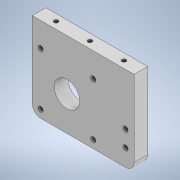
# Autodesk Inventor part: X-Axis_motor_plate
Saved by Autodesk Inventor 2021.3 (Build 253353000, 353)
## iProperties
Created: 2021-04-15
Part Number: X-Axis_motor_plate
Material: Generic
Document SubType Name: Modeling
Designer: Fabijan_Sven
Density: 1 g/cm^3
Appearance: Default
Author: Fabijan_Sven
Autodesk Inventor part; units mm, degrees
ref_plane "YZ Plane" through (0, 0, 0) normal (1, 0, 0) x (0, 1, 0)
ref_plane "XZ Plane" through (0, 0, 0) normal (0, 1, 0) x (-1, 0, 0)
ref_plane "XY Plane" through (0, 0, 0) normal (0, 0, 1) x (1, 0, 0)
sketch "Sketch1" plane through (0, 0, 0) normal (0, 1, 0) x (-1, 0, 0)
  line L0 (0, 0) -> (21.3426, 0)
  line L1 (21.3426, 0) -> (21.3426, -8)
  line L2 (21.3426, -8) -> (0, -8)
  line L3 (0, -8) -> (-38.6574, -8)
  line L4 (-38.6574, -8) -> (-38.6574, 0)
  line L5 (-38.6574, 0) -> (0, 0)
  dimension "d2" = 8
  dimension "d3" = 60
  dimension "d13" = 8
  constraints: 12 end point, 2 horizontal, 2 parallel, 2 perpendicular
  measures "d2" distance between parallel lines of L5 L3
  measures "d3" distance between parallel lines of L1 L4
  measures "d13" distance of L0.end L1.end
extrude "Extrusion1" add sketch "Sketch1" along normal blind 50
sketch "Sketch3" plane through (0, 0, 0) normal (0, 0, 1) x (1, 0, 0)
  circle A0 centre (-0.8634, 20.189) radius 7.5 projected
  line L0 (-17.3634, -0.311) -> (-21.3634, 3.689) projected
  line L1 (-17.3634, -0.311) -> (15.6366, -0.311) projected
  line L2 (19.6366, 3.689) -> (15.6366, -0.311) projected
  line L3 (19.6366, 3.689) -> (19.6366, 36.689) projected
  line L4 (15.6366, 40.689) -> (19.6366, 36.689) projected
  line L5 (15.6366, 40.689) -> (-17.3634, 40.689) projected
  line L6 (-21.3634, 36.689) -> (-17.3634, 40.689) projected
  line L7 (-21.3634, 36.689) -> (-21.3634, 3.689) projected
  circle A1 centre (-16.3634, 35.689) radius 1.5 projected
  circle A2 centre (14.6366, 4.689) radius 1.5 projected
  circle A3 centre (14.6366, 35.689) radius 1.5 projected
  circle A4 centre (-16.3634, 4.689) radius 1.5 projected
  circle A5 centre (33.6574, 10) radius 1.5
  circle A6 centre (33.6574, 19.5) radius 1.5
  line L8 (38.6574, 0) -> (38.6574, 50) projected
  line L9 (-21.3426, 0) -> (38.6574, 0) projected
  point P0 (0, 0)
  dimension "d6" = 5
  dimension "d7" = 5
  dimension "d8" = 3
  dimension "d9" = 3
  dimension "d11" = 9.5
  dimension "d12" = 10
  constraints: 2 centre point
  measures "d6" distance from line of L8 A5.centre
  measures "d7" distance from line of L8 A6.centre
  measures "d8" diameter of A6
  measures "d9" diameter of A5
  measures "d11" distance of A6.centre A5.centre
  measures "d12" distance from line of L9 A5.centre
extrude "Extrusion2" cut sketch "Sketch3" against normal blind 10 contours A0 | A1 | A2 | A3 | A4 | A5 | A6
fillet "Fillet1" radius 5 2 edges at (38.6574, 0, -4) (-21.3426, 0, -4)
sketch "Sketch4" plane through (0, 50, 0) normal (0, 1, 0) x (1, 0, 0)
  circle A0 centre (-11.3426, 2.5) radius 1.5 projected
  circle A1 centre (8.6574, 2.5) radius 1.5 projected
  circle A2 centre (28.6574, 2.5) radius 1.5 projected
  circle A3 centre (-11.3426, 4) radius 1.5
  circle A4 centre (8.6574, 4) radius 1.5
  circle A5 centre (28.6574, 4) radius 1.5
  line L0 (-25.013, 4) -> (50.4038, 4)
  line L1 (-21.3426, 8) -> (-21.3426, 0) projected
  line L2 (-21.3426, 0) -> (38.6574, 0) projected
  point P0 (0, 0)
  dimension "d21" = 3
  dimension "d22" = 10
  dimension "d23" = 20
  dimension "d24" = 20
  dimension "d25" = 4
  dimension "d26" = 3
  dimension "d27" = 3
  constraints: 3 centre point, 3 point on line, 2 end point, 1 horizontal
  measures "d21" diameter of A3
  measures "d22" distance from line of L1 A3.centre
  measures "d23" distance of A4.centre A3.centre
  measures "d24" distance of A5.centre A4.centre
  measures "d25" distance between parallel lines of L2 L0
  measures "d26" diameter of A4
  measures "d27" diameter of A5
hole "Hole1" at (-11.3426, 50, -4) at (8.6574, 50, -4) at (28.6574, 50, -4) direction (0, -1, 0) diameter 2.459 depth 20 tip angle 118 thread size "M3x0.5" class "6H" standard "ISO Metric profile"
body "Solid1"
